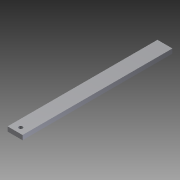
# Autodesk Inventor part: arm
Saved by Autodesk Inventor 2012 (Build 160160000, 160)
## iProperties
Created: 2014-03-21
Part Number: arm
Material: Default
Document SubType Name: Modeling
Designer: joe_000
Density: 1 g/cm^3
Author: joe_000
Autodesk Inventor part; units mm, degrees
ref_plane "YZ Plane" through (0, 0, 0) normal (1, 0, 0) x (0, 1, 0)
ref_plane "XZ Plane" through (0, 0, 0) normal (0, 1, 0) x (-1, 0, 0)
ref_plane "XY Plane" through (0, 0, 0) normal (0, 0, 1) x (1, 0, 0)
sketch "Sketch1" plane through (0, 0, 0) normal (0, 0, 1) x (1, 0, 0)
  line L0 (0, 0) -> (10, 0)
  line L1 (10, 0) -> (10, 100)
  line L2 (10, 100) -> (0, 100)
  line L3 (0, 100) -> (0, 0)
  dimension "d0" = 10
  dimension "d1" = 100
  constraints: 8 end point, 2 parallel, 1 horizontal, 1 perpendicular
  measures "d0" distance of L0.start L0.end
  measures "d1" distance of L0.end L1.end
extrude "Extrusion1" add sketch "Sketch1" along normal blind 3
sketch "Sketch2" plane through (0, 0, 3) normal (0, 0, 1) x (1, 0, 0)
  circle A0 centre (5, 3.75) radius 1.25
  line L0 (0, 0) -> (0, 100) projected
  line L1 (10, 0) -> (0, 0) projected
  dimension "d4" = 2.5
  dimension "d14" = 3.75
  dimension "d18" = 5
  constraints: 1 centre point
  measures "d4" diameter of A0
  measures "d14" distance from line of L1 A0.centre
  measures "d18" distance from line of L0 A0.centre
extrude "Extrusion4" cut sketch "Sketch2" against normal through all
equation "\"d4\" = centerHoleDia"
equation "\"centerHoleDia\" = 2.5"
body "Solid1"
